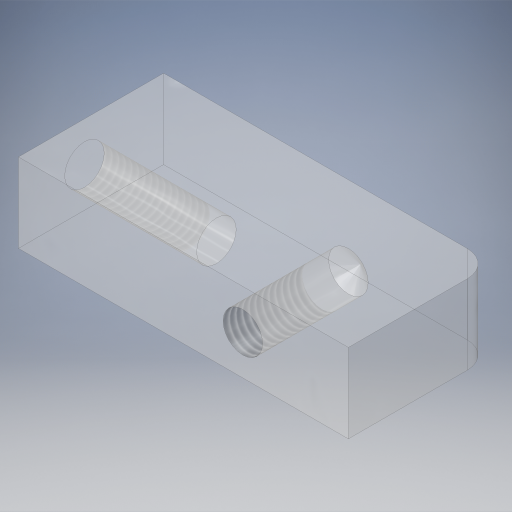
# Autodesk Inventor part: BT902_goteln20_23
Saved by Autodesk Inventor 2023 (Build 270158000, 158)
## iProperties
Company: HTBLA Kaindorf
RuleStatus: InUse
Created: 2023-01-10
Part Number: BT902_goteln20_23
Project: Zeichenmaschine_neu
Material: Acryl
Description: stepper_getriebe_winkel
Document SubType Name: Modeling
Designer: goteln20
Density: 1.188 g/cm^3
Appearance: Transparent - farblos
Mass: 1.79788 g
Surface Area: 11.4713 cm^2
Volume: 1.51337 cm^3
AfterDocNew0: iProperties-Editor_aufrufen
Author: eligo
Keywords: 23
Autodesk Inventor part; units mm, degrees
ref_plane "YZ Plane" through (0, 0, 0) normal (1, 0, 0) x (0, 1, 0)
ref_plane "XZ Plane" through (0, 0, 0) normal (0, 1, 0) x (-1, 0, 0)
ref_plane "XY Plane" through (0, 0, 0) normal (0, 0, 1) x (1, 0, 0)
sketch "Skizze3" plane through (0, 0, 0) normal (0, 0, 1) x (1, 0, 0)
  line L0 (0, 0) -> (-11, 0)
  line L1 (-11, 0) -> (-11, -25)
  line L2 (-11, -25) -> (0, -25)
  line L3 (0, -25) -> (0, 0)
  dimension "d4" = 11
  dimension "d5" = 25
  constraints: 8 end point, 2 parallel, 1 horizontal, 1 perpendicular
  measures "d4" distance of L1.end L2.end
  measures "d5" distance of L0.end L1.end
extrude "Extrusion3" add sketch "Skizze3" along normal blind 6
sketch "Skizze4" plane through (-11, -25, 0) normal (0, -1, 0) x (1, 0, 0)
  line L0 (11, 0) -> (11, 6) projected
  line L1 (0, 0) -> (0, 6) projected
  point P0 (6, 3)
  point P1 (0, 3)
  dimension "d8" = 5
  constraints: 1 horizontal alignment, 1 midpoint
  measures "d8" distance from line of point (6, 3) L0
hole "Bohrung1" at (-5, -25, 3) direction (0, 1, 0) diameter 3 depth 10 tip angle 118
thread "Gewinde1" size "M3x0.5" class "6H" standard "ISO Metric profile" length 8
sketch "Skizze5" plane through (0, -25, 0) normal (1, 0, 0) x (0, 0, -1)
  line L0 (0, 25) -> (-6, 25) projected
  line L1 (0, 0) -> (-6, 0) projected
  point P0 (-3, 17)
  point P1 (-3, 25)
  dimension "d18" = 17
  constraints: 1 midpoint, 1 vertical alignment
  measures "d18" distance from line of L1 point (-3, 17)
hole "Bohrung2" at (0, -8, 3) direction (-1, 0, 0) diameter 3 depth 8 tip angle 118
thread "Gewinde2" size "M3x0.5" class "6H" standard "ISO Metric profile" length 6
fillet "Rundung1" radius 2 1 edges at (-11, 0, 3)
